Autodesk Fusion 360 part; units mm, degrees
(part 2 of 5)
  line L70 (-24.2901, -31.3342) -> (-24.2626, -31.2045)
  spline S218 degree 3 poles (-24.2626, -31.2045) (-24.2478, -31.133) (-24.1584, -30.8424) (-24.0641, -30.5586) knots 0 0 0 0 1 1 1 1
  spline S219 degree 3 poles (-23.1509, -35.7407) (-21.6967, -38.062) (-19.505, -39.4527) (-18.2798, -38.8318) knots 0 0 0 0 1 1 1 1
  spline S220 degree 3 poles (-18.2798, -38.8318) (-17.8908, -38.6347) (-17.6834, -38.3768) (-18.0232, -38.5126) knots 0 0 0 0 1 1 1 1
  spline S221 degree 3 poles (-18.0232, -38.5126) (-19.0953, -38.9415) (-20.3855, -38.1958) (-23.002, -35.6358) knots 0 0 0 0 1 1 1 1
  spline S222 degree 3 poles (-23.002, -35.6358) (-23.4422, -35.2048) (-23.4732, -35.2265) (-23.1509, -35.7407) knots 0 0 0 0 1 1 1 1
  spline S223 degree 3 poles (-20.8842, -40.3996) (-20.7556, -40.3996) (-20.6902, -40.5127) (-20.7714, -40.5939) knots 0 0 0 0 1 1 1 1
  spline S224 degree 3 poles (-20.7714, -40.5939) (-20.8663, -40.6892) (-21.0022, -40.6311) (-20.9874, -40.5014) knots 0 0 0 0 1 1 1 1
  spline S225 degree 3 poles (-20.9874, -40.5014) (-20.9781, -40.423) (-20.9547, -40.3996) (-20.8842, -40.3996) knots 0 0 0 0 1 1 1 1
  spline S226 degree 3 poles (-15.859, -39.81) (-15.7052, -39.9693) (-15.4972, -40.2273) (-15.3967, -40.3834) knots 0 0 0 0 1 1 1 1
  spline S227 degree 3 poles (-15.3967, -40.3834) (-15.0184, -40.9719) (-14.932, -41.0844) (-14.7484, -41.2302) knots 0 0 0 0 1 1 1 1
  spline S228 degree 3 poles (-14.7484, -41.2302) (-14.5557, -41.3833) (-14.2304, -41.5653) (-14.1499, -41.5653) knots 0 0 0 0 1 1 1 1
  spline S229 degree 3 poles (-14.1499, -41.5653) (-14.1251, -41.5653) (-14.2407, -41.4236) (-14.4068, -41.2499) knots 0 0 0 0 1 1 1 1
  spline S230 degree 3 poles (-14.4068, -41.2499) (-14.5726, -41.0765) (-14.7934, -40.7972) (-14.8973, -40.629) knots 0 0 0 0 1 1 1 1
  spline S231 degree 3 poles (-14.8973, -40.629) (-15.2719, -40.0226) (-15.5315, -39.7523) (-15.9388, -39.5452) knots 0 0 0 0 1 1 1 1
  spline S232 degree 3 poles (-15.9388, -39.5452) (-16.2274, -39.3987) (-16.214, -39.443) (-15.859, -39.81) knots 0 0 0 0 1 1 1 1
  spline S233 degree 3 poles (-15.6155, -38.9729) (-15.2839, -39.2931) (-14.9551, -39.4286) (-14.3803, -39.4819) knots 0 0 0 0 1 1 1 1
  spline S234 degree 3 poles (-14.3803, -39.4819) (-13.7203, -39.5431) (-12.3448, -39.3147) (-12.2268, -39.1245) knots 0 0 0 0 1 1 1 1
  spline S235 degree 3 poles (-12.2268, -39.1245) (-12.2185, -39.1111) (-12.7586, -39.106) (-13.4265, -39.1125) knots 0 0 0 0 1 1 1 1
  spline S236 degree 3 poles (-13.4265, -39.1125) (-14.7814, -39.1263) (-14.9286, -39.1111) (-15.3916, -38.9072) knots 0 0 0 0 1 1 1 1
  spline S237 degree 3 poles (-15.3916, -38.9072) (-15.5622, -38.8318) (-15.7231, -38.7613) (-15.7493, -38.7496) knots 0 0 0 0 1 1 1 1
  spline S238 degree 3 poles (-15.7493, -38.7496) (-15.849, -38.7066) (-15.7905, -38.8036) (-15.6155, -38.9729) knots 0 0 0 0 1 1 1 1
  spline S239 degree 3 poles (-13.7519, -74.1202) (-12.6942, -87.0541) (-11.8189, -97.6776) (-11.8061, -97.7278) knots 0 0 0 0 1 1 1 1
  spline S240 degree 3 poles (-11.8061, -97.7278) (-11.7607, -97.9101) (-11.4151, -97.9504) (-11.326, -97.7842) knots 0 0 0 0 1 1 1 1
  spline S241 degree 3 poles (-11.326, -97.7842) (-11.2393, -97.6222) (-11.2764, -47.9849) (-11.3638, -47.8422) knots 0 0 0 0 1 1 1 1
  spline S242 degree 3 poles (-11.3638, -47.8422) (-11.5103, -47.6017) (-11.8199, -47.4865) (-12.0768, -47.5766) knots 0 0 0 0 1 1 1 1
  spline S243 degree 3 poles (-12.0768, -47.5766) (-12.3517, -47.6733) (-15.5192, -49.7374) (-15.6048, -49.8756) knots 0 0 0 0 1 1 1 1
  spline S244 degree 3 poles (-15.6048, -49.8756) (-15.7235, -50.0676) (-15.7985, -49.0845) (-13.7519, -74.1202) knots 0 0 0 0 1 1 1 1
  spline S245 degree 3 poles (-15.6055, -12.3577) (-15.59, -12.4261) (-15.5364, -12.5335) (-15.4865, -12.5964) knots 0 0 0 0 1 1 1 1
  spline S246 degree 3 poles (-15.4865, -12.5964) (-15.3713, -12.7416) (-12.158, -14.8015) (-11.9657, -14.8538) knots 0 0 0 0 1 1 1 1
  spline S247 degree 3 poles (-11.9657, -14.8538) (-11.6961, -14.9264) (-11.3941, -14.7857) (-11.273, -14.5312) knots 0 0 0 0 1 1 1 1
  spline S248 degree 3 poles (-11.273, -14.5312) (-11.2159, -14.4104) (-11.2111, -12.4203) (-11.2111, 10.4615) knots 0 0 0 0 1 1 1 1
  line L71 (-11.2111, 10.4615) -> (-11.2111, 35.3228)
  line L72 (-11.2111, 35.3228) -> (-11.3115, 35.4023)
  spline S249 degree 3 poles (-11.3115, 35.4023) (-11.4347, 35.4989) (-11.5578, 35.5031) (-11.6675, 35.4143) knots 0 0 0 0 1 1 1 1
  spline S250 degree 3 poles (-11.6675, 35.4143) (-11.748, 35.349) (-11.7989, 34.7477) (-13.6755, 11.729) knots 0 0 0 0 1 1 1 1
  spline S251 degree 3 poles (-13.6755, 11.729) (-14.7346, -1.2609) (-15.6082, -11.9666) (-15.6172, -12.0612) knots 0 0 0 0 1 1 1 1
  spline S252 degree 3 poles (-15.6172, -12.0612) (-15.6261, -12.1558) (-15.6206, -12.2892) (-15.6055, -12.3577) knots 0 0 0 0 1 1 1 1
  spline S253 degree 3 poles (-15.1442, -35.3867) (-14.6259, -35.8559) (-13.8018, -36.1269) (-13.1434, -36.0447) knots 0 0 0 0 1 1 1 1
  spline S254 degree 3 poles (-13.1434, -36.0447) (-12.8686, -36.0103) (-12.8755, -35.9856) (-13.1888, -35.8765) knots 0 0 0 0 1 1 1 1
  spline S255 degree 3 poles (-13.1888, -35.8765) (-13.4503, -35.7854) (-15.2412, -35.1494) (-15.329, -35.1164) knots 0 0 0 0 1 1 1 1
  spline S256 degree 3 poles (-15.329, -35.1164) (-15.4404, -35.0744) (-15.3609, -35.191) (-15.1442, -35.3867) knots 0 0 0 0 1 1 1 1
  spline S257 degree 3 poles (-10.2752, -41.426) (-10.171, -41.0755) (-9.569, -40.3411) (-9.3878, -40.3432) knots 0 0 0 0 1 1 1 1
  spline S258 degree 3 poles (-9.3878, -40.3432) (-9.0524, -40.3473) (-8.8275, -40.6087) (-8.8797, -40.9341) knots 0 0 0 0 1 1 1 1
  spline S259 degree 3 poles (-8.8797, -40.9341) (-8.9637, -41.4597) (-9.1202, -41.6488) (-9.5436, -41.7376) knots 0 0 0 0 1 1 1 1
  spline S260 degree 3 poles (-9.5436, -41.7376) (-9.686, -41.7675) (-9.8573, -41.8256) (-9.9243, -41.8673) knots 0 0 0 0 1 1 1 1
  spline S261 degree 3 poles (-9.9243, -41.8673) (-10.3061, -42.1032) (-10.43, -41.9477) (-10.2752, -41.426) knots 0 0 0 0 1 1 1 1
  spline S262 degree 3 poles (-4.9222, -79.0378) (-4.4427, -81.601) (-2.4986, -83.2055) (0.1206, -83.1997) knots 0 0 0 0 1 1 1 1
  spline S263 degree 3 poles (0.1206, -83.1997) (3.6706, -83.1918) (5.9848, -79.9675) (4.9739, -76.4378) knots 0 0 0 0 1 1 1 1
  spline S264 degree 3 poles (4.9739, -76.4378) (3.682, -71.9251) (-2.9984, -71.6857) (-4.6573, -76.0925) knots 0 0 0 0 1 1 1 1
  spline S265 degree 3 poles (-4.6573, -76.0925) (-4.9524, -76.8767) (-5.0738, -78.2264) (-4.9222, -79.0378) knots 0 0 0 0 1 1 1 1
  spline S266 degree 3 poles (-4.9242, -57.9033) (-4.4138, -60.7987) (-1.6762, -62.6382) (1.1996, -62.0184) knots 0 0 0 0 1 1 1 1
  spline S267 degree 3 poles (1.1996, -62.0184) (5.118, -61.174) (6.5392, -56.3479) (3.7927, -53.212) knots 0 0 0 0 1 1 1 1
  spline S268 degree 3 poles (3.7927, -53.212) (3.6317, -53.028) (3.479, -52.8777) (3.4529, -52.8777) knots 0 0 0 0 1 1 1 1
  spline S269 degree 3 poles (3.4529, -52.8777) (3.4102, -52.8777) (3.1217, -53.1625) (2.2081, -54.1063) knots 0 0 0 0 1 1 1 1
  line L73 (2.2081, -54.1063) -> (1.8882, -54.4365)
  line L74 (1.8882, -54.4365) -> (2.0781, -54.6649)
  spline S270 degree 3 poles (2.0781, -54.6649) (3.8804, -56.8305) (2.7553, -59.6901) (0.1014, -59.6901) knots 0 0 0 0 1 1 1 1
  spline S271 degree 3 poles (0.1014, -59.6901) (-2.5523, -59.6901) (-3.6774, -56.8305) (-1.8757, -54.6656) knots 0 0 0 0 1 1 1 1
  line L75 (-1.8757, -54.6656) -> (-1.6865, -54.4379)
  line L76 (-1.6865, -54.4379) -> (-1.798, -54.3172)
  spline S272 degree 3 poles (-1.798, -54.3172) (-1.8592, -54.2504) (-2.2094, -53.8803) (-2.576, -53.4944) knots 0 0 0 0 1 1 1 1
  line L77 (-2.576, -53.4944) -> (-3.2426, -52.7924)
  line L78 (-3.2426, -52.7924) -> (-3.537, -53.1061)
  spline S273 degree 3 poles (-3.537, -53.1061) (-4.1995, -53.8119) (-4.6312, -54.613) (-4.8554, -55.553) knots 0 0 0 0 1 1 1 1
  spline S274 degree 3 poles (-4.8554, -55.553) (-4.9762, -56.06) (-5.0154, -57.3877) (-4.9242, -57.9033) knots 0 0 0 0 1 1 1 1
  spline S275 degree 3 poles (-4.9222, -38.4889) (-4.4427, -41.0521) (-2.4986, -42.6566) (0.1206, -42.6508) knots 0 0 0 0 1 1 1 1
  spline S276 degree 3 poles (0.1206, -42.6508) (3.6706, -42.6429) (5.9848, -39.4186) (4.9739, -35.8889) knots 0 0 0 0 1 1 1 1
  spline S277 degree 3 poles (4.9739, -35.8889) (3.682, -31.3762) (-2.9984, -31.1371) (-4.6573, -35.5439) knots 0 0 0 0 1 1 1 1
  spline S278 degree 3 poles (-4.6573, -35.5439) (-4.9524, -36.3278) (-5.0738, -37.6775) (-4.9222, -38.4889) knots 0 0 0 0 1 1 1 1
  spline S279 degree 3 poles (-4.9222, -15.6346) (-4.4427, -18.1978) (-2.4986, -19.8027) (0.1206, -19.7968) knots 0 0 0 0 1 1 1 1
  spline S280 degree 3 poles (0.1206, -19.7968) (3.6706, -19.7889) (5.9848, -16.5646) (4.9739, -13.0346) knots 0 0 0 0 1 1 1 1
  spline S281 degree 3 poles (4.9739, -13.0346) (3.682, -8.5222) (-2.9984, -8.2828) (-4.6573, -12.6896) knots 0 0 0 0 1 1 1 1
  spline S282 degree 3 poles (-4.6573, -12.6896) (-4.9524, -13.4738) (-5.0738, -14.8235) (-4.9222, -15.6346) knots 0 0 0 0 1 1 1 1
  spline S283 degree 3 poles (-4.9222, 3.474) (-4.4427, 0.9108) (-2.4986, -0.6937) (0.1206, -0.6879) knots 0 0 0 0 1 1 1 1
  spline S284 degree 3 poles (0.1206, -0.6879) (3.6706, -0.68) (5.9848, 2.5443) (4.9739, 6.074) knots 0 0 0 0 1 1 1 1
  spline S285 degree 3 poles (4.9739, 6.074) (3.682, 10.5867) (-2.9984, 10.8258) (-4.6573, 6.419) knots 0 0 0 0 1 1 1 1
  spline S286 degree 3 poles (-4.6573, 6.419) (-4.9524, 5.6351) (-5.0738, 4.2854) (-4.9222, 3.474) knots 0 0 0 0 1 1 1 1
  spline S287 degree 3 poles (-4.9242, 24.6085) (-4.4138, 21.7131) (-1.6762, 19.8736) (1.1996, 20.4934) knots 0 0 0 0 1 1 1 1
  spline S288 degree 3 poles (1.1996, 20.4934) (5.118, 21.3378) (6.5392, 26.1639) (3.7927, 29.2998) knots 0 0 0 0 1 1 1 1
  spline S289 degree 3 poles (3.7927, 29.2998) (3.6317, 29.4835) (3.479, 29.6341) (3.4529, 29.6341) knots 0 0 0 0 1 1 1 1
  spline S290 degree 3 poles (3.4529, 29.6341) (3.4102, 29.6341) (3.1217, 29.3493) (2.2081, 28.4055) knots 0 0 0 0 1 1 1 1
  line L79 (2.2081, 28.4055) -> (1.8882, 28.0753)
  line L80 (1.8882, 28.0753) -> (2.0781, 27.8469)
  spline S291 degree 3 poles (2.0781, 27.8469) (3.8804, 25.6813) (2.7553, 22.8217) (0.1014, 22.8217) knots 0 0 0 0 1 1 1 1
  spline S292 degree 3 poles (0.1014, 22.8217) (-2.5523, 22.8217) (-3.6774, 25.6813) (-1.8757, 27.8462) knots 0 0 0 0 1 1 1 1
  line L81 (-1.8757, 27.8462) -> (-1.6865, 28.0739)
  line L82 (-1.6865, 28.0739) -> (-1.798, 28.1947)
  spline S293 degree 3 poles (-1.798, 28.1947) (-1.8592, 28.261) (-2.2094, 28.6315) (-2.576, 29.0174) knots 0 0 0 0 1 1 1 1
  line L83 (-2.576, 29.0174) -> (-3.2426, 29.7194)
  line L84 (-3.2426, 29.7194) -> (-3.537, 29.4057)
  spline S294 degree 3 poles (-3.537, 29.4057) (-4.1995, 28.6999) (-4.6312, 27.8988) (-4.8554, 26.9588) knots 0 0 0 0 1 1 1 1
  spline S295 degree 3 poles (-4.8554, 26.9588) (-4.9762, 26.4518) (-5.0154, 25.1241) (-4.9242, 24.6085) knots 0 0 0 0 1 1 1 1
  spline S296 degree 3 poles (-4.9252, 32.6341) (-4.5713, 31.0117) (-3.1164, 29.9402) (-1.5187, 30.126) knots 0 0 0 0 1 1 1 1
  spline S297 degree 3 poles (-1.5187, 30.126) (-0.1704, 30.2828) (0.499, 30.9728) (1.1549, 32.8828) knots 0 0 0 0 1 1 1 1
  spline S298 degree 3 poles (1.1549, 32.8828) (1.6144, 34.2208) (1.9742, 34.5482) (2.6239, 34.2194) knots 0 0 0 0 1 1 1 1
  spline S299 degree 3 poles (2.6239, 34.2194) (3.3851, 33.8342) (3.0343, 32.424) (2.1768, 32.424) knots 0 0 0 0 1 1 1 1
  line L85 (2.1768, 32.424) -> (2.0506, 32.424)
  line L86 (2.0506, 32.424) -> (2.0506, 31.2545)
  line L87 (2.0506, 31.2545) -> (2.0506, 30.085)
  line L88 (2.0506, 30.085) -> (2.3275, 30.1108)
  spline S300 degree 3 poles (2.3275, 30.1108) (4.2423, 30.2897) (5.3419, 31.6934) (5.1765, 33.7479) knots 0 0 0 0 1 1 1 1
  spline S301 degree 3 poles (5.1765, 33.7479) (4.9292, 36.8191) (0.8178, 37.7501) (-0.5377, 35.0418) knots 0 0 0 0 1 1 1 1
  spline S302 degree 3 poles (-0.5377, 35.0418) (-0.6794, 34.7581) (-0.8094, 34.3948) (-0.9821, 33.7998) knots 0 0 0 0 1 1 1 1
  spline S303 degree 3 poles (-0.9821, 33.7998) (-1.2934, 32.7256) (-1.4929, 32.4529) (-1.9634, 32.4563) knots 0 0 0 0 1 1 1 1
  spline S304 degree 3 poles (-1.9634, 32.4563) (-3.0624, 32.4649) (-3.1387, 34.2094) (-2.0484, 34.3911) knots 0 0 0 0 1 1 1 1
  line L89 (-2.0484, 34.3911) -> (-1.886, 34.4179)
  line L90 (-1.886, 34.4179) -> (-1.886, 35.5285)
  line L91 (-1.886, 35.5285) -> (-1.886, 36.6388)
  line L92 (-1.886, 36.6388) -> (-2.1454, 36.6147)
  spline S305 degree 3 poles (-2.1454, 36.6147) (-4.129, 36.4304) (-5.3669, 34.658) (-4.9252, 32.6341) knots 0 0 0 0 1 1 1 1
  line L93 (0.1189, -99.0827) -> (4.9168, -99.0827)
  line L94 (4.9168, -99.0827) -> (4.9161, -97.0478)
  spline S306 degree 3 poles (4.9161, -97.0478) (4.9157, -95.9282) (4.8989, -94.8097) (4.8783, -94.5617) knots 0 0 0 0 1 1 1 1
  spline S307 degree 3 poles (4.8783, -94.5617) (4.6598, -91.9245) (1.8174, -91.0416) (0.1781, -93.1012) knots 0 0 0 0 1 1 1 1
  line L95 (0.1781, -93.1012) -> (-0.017, -93.3468)
  line L96 (-0.017, -93.3468) -> (-0.3303, -93.0304)
  spline S308 degree 3 poles (-0.3303, -93.0304) (-1.5407, -91.8086) (-3.7197, -92.2936) (-4.4275, -93.9425) knots 0 0 0 0 1 1 1 1
  spline S309 degree 3 poles (-4.4275, -93.9425) (-4.6642, -94.4932) (-4.6521, -94.3474) (-4.6662, -96.8184) knots 0 0 0 0 1 1 1 1
  line L97 (-4.6662, -96.8184) -> (-4.6793, -99.0827)
  line L98 (-4.6793, -99.0827) -> (0.1189, -99.0827)
  line L99 (0.1206, -91.3629) -> (4.9168, -91.3629)
  line L100 (4.9168, -91.3629) -> (4.9168, -90.1786)
  line L101 (4.9168, -90.1786) -> (4.9168, -88.994)
  line L102 (4.9168, -88.994) -> (3.1726, -88.984)
  line L103 (3.1726, -88.984) -> (1.428, -88.9741)
  line L104 (1.428, -88.9741) -> (3.1629, -87.7854)
  line L105 (3.1629, -87.7854) -> (4.8979, -86.5963)
  line L106 (4.8979, -86.5963) -> (4.9078, -85.1197)
  spline S310 degree 3 poles (4.9078, -85.1197) (4.914, -84.1972) (4.904, -83.6427) (4.881, -83.6427) knots 0 0 0 0 1 1 1 1
  spline S311 degree 3 poles (4.881, -83.6427) (4.8611, -83.6427) (4.0655, -84.2102) (3.1131, -84.9033) knots 0 0 0 0 1 1 1 1
  spline S312 degree 3 poles (3.1131, -84.9033) (2.161, -85.5967) (1.3719, -86.1643) (1.3602, -86.1646) knots 0 0 0 0 1 1 1 1
  spline S313 degree 3 poles (1.3602, -86.1646) (1.3486, -86.165) (1.3162, -86.0762) (1.2884, -85.9675) knots 0 0 0 0 1 1 1 1
  spline S314 degree 3 poles (1.2884, -85.9675) (1.0514, -85.0433) (0.2806, -84.2983) (-0.6908, -84.0544) knots 0 0 0 0 1 1 1 1
  spline S315 degree 3 poles (-0.6908, -84.0544) (-2.3731, -83.6327) (-3.9494, -84.418) (-4.4654, -85.9352) knots 0 0 0 0 1 1 1 1
  spline S316 degree 3 poles (-4.4654, -85.9352) (-4.6683, -86.532) (-4.6759, -86.6441) (-4.6759, -89.0931) knots 0 0 0 0 1 1 1 1
  line L107 (-4.6759, -89.0931) -> (-4.6759, -91.3629)
  line L108 (-4.6759, -91.3629) -> (0.1206, -91.3629)
  line L109 (0.1206, -71.7572) -> (4.9168, -71.7572)
  line L110 (4.9168, -71.7572) -> (4.9168, -70.5726)
  line L111 (4.9168, -70.5726) -> (4.9168, -69.3881)
  line L112 (4.9168, -69.3881) -> (2.1183, -69.3784)
  line L113 (2.1183, -69.3784) -> (-0.6805, -69.3684)
  line L114 (-0.6805, -69.3684) -> (2.1183, -67.5348)
  line L115 (2.1183, -67.5348) -> (4.9168, -65.7008)
  line L116 (4.9168, -65.7008) -> (4.9168, -64.4677)
  line L117 (4.9168, -64.4677) -> (4.9168, -63.2346)
  line L118 (4.9168, -63.2346) -> (0.1206, -63.2346)
  line L119 (0.1206, -63.2346) -> (-4.6759, -63.2346)
  line L120 (-4.6759, -63.2346) -> (-4.6759, -64.4192)
  line L121 (-4.6759, -64.4192) -> (-4.6759, -65.6038)
  line L122 (-4.6759, -65.6038) -> (-1.8964, -65.6135)
  line L123 (-1.8964, -65.6135) -> (0.8832, -65.6234)
  line L124 (0.8832, -65.6234) -> (-1.8964, -67.4364)
  line L125 (-1.8964, -67.4364) -> (-4.6759, -69.2494)
  line L126 (-4.6759, -69.2494) -> (-4.6759, -70.5032)
  line L127 (-4.6759, -70.5032) -> (-4.6759, -71.7572)
  line L128 (-4.6759, -71.7572) -> (0.1206, -71.7572)
  line L129 (0.1206, -52.1898) -> (4.9168, -52.1898)
  line L130 (4.9168, -52.1898) -> (4.9168, -51.0052)
  line L131 (4.9168, -51.0052) -> (4.9168, -49.8203)
  line L132 (4.9168, -49.8203) -> (3.0061, -49.8203)
  line L133 (3.0061, -49.8203) -> (1.0951, -49.8203)
  line L134 (1.0951, -49.8203) -> (1.0951, -47.9667)
  line L135 (1.0951, -47.9667) -> (1.0951, -46.1131)
  line L136 (1.0951, -46.1131) -> (3.0061, -46.1131)
  line L137 (3.0061, -46.1131) -> (4.9168, -46.1131)
  line L138 (4.9168, -46.1131) -> (4.9168, -44.9474)
  line L139 (4.9168, -44.9474) -> (4.9168, -43.7821)
  line L140 (4.9168, -43.7821) -> (0.1206, -43.7821)
  line L141 (0.1206, -43.7821) -> (-4.6759, -43.7821)
  line L142 (-4.6759, -43.7821) -> (-4.6759, -44.9474)
  line L143 (-4.6759, -44.9474) -> (-4.6759, -46.1131)
  line L144 (-4.6759, -46.1131) -> (-2.803, -46.1131)
  line L145 (-2.803, -46.1131) -> (-0.9305, -46.1131)
  line L146 (-0.9305, -46.1131) -> (-0.9305, -47.9667)
  line L147 (-0.9305, -47.9667) -> (-0.9305, -49.8203)
  line L148 (-0.9305, -49.8203) -> (-2.803, -49.8203)
  line L149 (-2.803, -49.8203) -> (-4.6759, -49.8203)
  line L150 (-4.6759, -49.8203) -> (-4.6759, -51.0052)
  line L151 (-4.6759, -51.0052) -> (-4.6759, -52.1898)
  line L152 (-4.6759, -52.1898) -> (0.1206, -52.1898)
  line L153 (0.1206, -27.96) -> (4.9168, -27.96)
  line L154 (4.9168, -27.96) -> (4.9168, -26.7754)
  line L155 (4.9168, -26.7754) -> (4.9168, -25.5912)
  line L156 (4.9168, -25.5912) -> (3.1726, -25.5812)
  line L157 (3.1726, -25.5812) -> (1.428, -25.5712)
  line L158 (1.428, -25.5712) -> (3.1629, -24.3821)
  line L159 (3.1629, -24.3821) -> (4.8979, -23.1934)
  line L160 (4.8979, -23.1934) -> (4.9078, -21.7165)
  spline S317 degree 3 poles (4.9078, -21.7165) (4.914, -20.7943) (4.904, -20.2398) (4.881, -20.2398) knots 0 0 0 0 1 1 1 1
  spline S318 degree 3 poles (4.881, -20.2398) (4.8611, -20.2398) (4.0655, -20.807) (3.1131, -21.5005) knots 0 0 0 0 1 1 1 1
  spline S319 degree 3 poles (3.1131, -21.5005) (2.161, -22.1935) (1.3719, -22.7611) (1.3602, -22.7614) knots 0 0 0 0 1 1 1 1
  spline S320 degree 3 poles (1.3602, -22.7614) (1.3486, -22.7621) (1.3162, -22.6734) (1.2884, -22.5647) knots 0 0 0 0 1 1 1 1
  spline S321 degree 3 poles (1.2884, -22.5647) (1.0514, -21.6404) (0.2806, -20.8951) (-0.6908, -20.6516) knots 0 0 0 0 1 1 1 1
  spline S322 degree 3 poles (-0.6908, -20.6516) (-2.3731, -20.2295) (-3.9494, -21.0151) (-4.4654, -22.5323) knots 0 0 0 0 1 1 1 1
  spline S323 degree 3 poles (-4.4654, -22.5323) (-4.6683, -23.1291) (-4.6759, -23.2409) (-4.6759, -25.6902) knots 0 0 0 0 1 1 1 1
  line L161 (-4.6759, -25.6902) -> (-4.6759, -27.96)
  line L162 (-4.6759, -27.96) -> (0.1206, -27.96)
  line L163 (0.1189, -8.3544) -> (4.9168, -8.3544)
  line L164 (4.9168, -8.3544) -> (4.9161, -6.3192)
  spline S324 degree 3 poles (4.9161, -6.3192) (4.9157, -5.1999) (4.8989, -4.081) (4.8783, -3.833) knots 0 0 0 0 1 1 1 1
  spline S325 degree 3 poles (4.8783, -3.833) (4.6598, -1.1959) (1.8174, -0.313) (0.1781, -2.3729) knots 0 0 0 0 1 1 1 1
  line L165 (0.1781, -2.3729) -> (-0.017, -2.6182)
  line L166 (-0.017, -2.6182) -> (-0.3303, -2.3017)
  spline S326 degree 3 poles (-0.3303, -2.3017) (-1.5407, -1.08) (-3.7197, -1.565) (-4.4275, -3.2139) knots 0 0 0 0 1 1 1 1
  spline S327 degree 3 poles (-4.4275, -3.2139) (-4.6642, -3.7646) (-4.6521, -3.6191) (-4.6662, -6.0897) knots 0 0 0 0 1 1 1 1
  line L167 (-4.6662, -6.0897) -> (-4.6793, -8.3544)
  line L168 (-4.6793, -8.3544) -> (0.1189, -8.3544)
  line L169 (-3.644, 9.6464) -> (-2.6121, 9.6464)
  line L170 (-2.6121, 9.6464) -> (-2.6121, 10.7164)
  line L171 (-2.6121, 10.7164) -> (-2.6121, 11.7865)
  line L172 (-2.6121, 11.7865) -> (1.1525, 11.7865)
  line L173 (1.1525, 11.7865) -> (4.9168, 11.7865)
  line L174 (4.9168, 11.7865) -> (4.9168, 12.9711)
  line L175 (4.9168, 12.9711) -> (4.9168, 14.156)
  line L176 (4.9168, 14.156) -> (1.1525, 14.156)
  line L177 (1.1525, 14.156) -> (-2.6121, 14.156)
  line L178 (-2.6121, 14.156) -> (-2.6121, 15.2453)
  line L179 (-2.6121, 15.2453) -> (-2.6121, 16.3343)
  line L180 (-2.6121, 16.3343) -> (-3.644, 16.3343)
  line L181 (-3.644, 16.3343) -> (-4.6759, 16.3343)
  line L182 (-4.6759, 16.3343) -> (-4.6759, 12.9903)
  line L183 (-4.6759, 12.9903) -> (-4.6759, 9.6464)
  line L184 (-4.6759, 9.6464) -> (-3.644, 9.6464)
  line L185 (0.1206, 16.9458) -> (4.9168, 16.9458)
  line L186 (4.9168, 16.9458) -> (4.9168, 18.1304)
  line L187 (4.9168, 18.1304) -> (4.9168, 19.3154)
  line L188 (4.9168, 19.3154) -> (0.1206, 19.3154)
  line L189 (0.1206, 19.3154) -> (-4.6759, 19.3154)
  line L190 (-4.6759, 19.3154) -> (-4.6759, 18.1304)
  line L191 (-4.6759, 18.1304) -> (-4.6759, 16.9458)
  line L192 (-4.6759, 16.9458) -> (0.1206, 16.9458)
  spline S328 degree 3 poles (-4.4272, -77.1529) (-3.5357, -72.5222) (3.3672, -72.2945) (4.5343, -76.8571) knots 0 0 0 0 1 1 1 1
  spline S329 degree 3 poles (4.5343, -76.8571) (5.2993, -79.8489) (3.1846, -82.5778) (0.1014, -82.5778) knots 0 0 0 0 1 1 1 1
  spline S330 degree 3 poles (0.1014, -82.5778) (-2.8794, -82.5778) (-4.9861, -80.0545) (-4.4272, -77.1529) knots 0 0 0 0 1 1 1 1
  spline S331 degree 3 poles (-4.4833, -56.32) (-4.3832, -55.3449) (-4.012, -54.4472) (-3.45, -53.8205) knots 0 0 0 0 1 1 1 1
  line L193 (-3.45, -53.8205) -> (-3.2502, -53.5976)
  line L194 (-3.2502, -53.5976) -> (-2.8202, -54.0262)
  line L195 (-2.8202, -54.0262) -> (-2.3903, -54.4551)
  line L196 (-2.3903, -54.4551) -> (-2.5193, -54.6346)
  spline S332 degree 3 poles (-2.5193, -54.6346) (-3.4844, -55.9781) (-3.4603, -58.0254) (-2.4656, -59.2076) knots 0 0 0 0 1 1 1 1
  spline S333 degree 3 poles (-2.4656, -59.2076) (-1.1933, -60.7193) (1.396, -60.7193) (2.6683, -59.2076) knots 0 0 0 0 1 1 1 1
  spline S334 degree 3 poles (2.6683, -59.2076) (3.6589, -58.0305) (3.6913, -55.9551) (2.7385, -54.6893) knots 0 0 0 0 1 1 1 1
  line L197 (2.7385, -54.6893) -> (2.592, -54.4943)
  line L198 (2.592, -54.4943) -> (3.0309, -54.0589)
  line L199 (3.0309, -54.0589) -> (3.4697, -53.6231)
  line L200 (3.4697, -53.6231) -> (3.6053, -53.7758)
  spline S335 degree 3 poles (3.6053, -53.7758) (5.6553, -56.0927) (4.7868, -59.9516) (1.9491, -61.1327) knots 0 0 0 0 1 1 1 1
  spline S336 degree 3 poles (1.9491, -61.1327) (-1.4014, -62.5275) (-4.8551, -59.9436) (-4.4833, -56.32) knots 0 0 0 0 1 1 1 1
  spline S337 degree 3 poles (-4.4272, -36.604) (-3.5357, -31.9733) (3.3672, -31.7456) (4.5343, -36.3082) knots 0 0 0 0 1 1 1 1
  spline S338 degree 3 poles (4.5343, -36.3082) (5.2993, -39.3) (3.1846, -42.0289) (0.1014, -42.0289) knots 0 0 0 0 1 1 1 1
  spline S339 degree 3 poles (0.1014, -42.0289) (-2.8794, -42.0289) (-4.9861, -39.5056) (-4.4272, -36.604) knots 0 0 0 0 1 1 1 1
  spline S340 degree 3 poles (-4.4272, -13.75) (-3.5357, -9.1193) (3.3672, -8.8916) (4.5343, -13.4542) knots 0 0 0 0 1 1 1 1
  spline S341 degree 3 poles (4.5343, -13.4542) (5.2993, -16.4456) (3.1846, -19.175) (0.1014, -19.175) knots 0 0 0 0 1 1 1 1
  spline S342 degree 3 poles (0.1014, -19.175) (-2.8794, -19.175) (-4.9861, -16.6517) (-4.4272, -13.75) knots 0 0 0 0 1 1 1 1
  spline S343 degree 3 poles (-4.4272, 5.3589) (-3.5357, 9.9896) (3.3672, 10.2173) (4.5343, 5.6547) knots 0 0 0 0 1 1 1 1
  spline S344 degree 3 poles (4.5343, 5.6547) (5.2993, 2.663) (3.1846, -0.066) (0.1014, -0.066) knots 0 0 0 0 1 1 1 1
  spline S345 degree 3 poles (0.1014, -0.066) (-2.8794, -0.066) (-4.9861, 2.4573) (-4.4272, 5.3589) knots 0 0 0 0 1 1 1 1
  spline S346 degree 3 poles (-4.4833, 26.1914) (-4.3832, 27.1669) (-4.012, 28.0646) (-3.45, 28.6913) knots 0 0 0 0 1 1 1 1
  line L201 (-3.45, 28.6913) -> (-3.2502, 28.9142)
  line L202 (-3.2502, 28.9142) -> (-2.8202, 28.4856)
  line L203 (-2.8202, 28.4856) -> (-2.3903, 28.0567)
  line L204 (-2.3903, 28.0567) -> (-2.5193, 27.8772)
  spline S347 degree 3 poles (-2.5193, 27.8772) (-3.4844, 26.5337) (-3.4603, 24.4864) (-2.4656, 23.3042) knots 0 0 0 0 1 1 1 1
  spline S348 degree 3 poles (-2.4656, 23.3042) (-1.1933, 21.7926) (1.396, 21.7926) (2.6683, 23.3042) knots 0 0 0 0 1 1 1 1
  spline S349 degree 3 poles (2.6683, 23.3042) (3.6589, 24.4813) (3.6913, 26.5567) (2.7385, 27.8225) knots 0 0 0 0 1 1 1 1
  line L205 (2.7385, 27.8225) -> (2.592, 28.0175)
  line L206 (2.592, 28.0175) -> (3.0309, 28.453)
  line L207 (3.0309, 28.453) -> (3.4697, 28.8887)
  line L208 (3.4697, 28.8887) -> (3.6053, 28.736)
  spline S350 degree 3 poles (3.6053, 28.736) (5.6553, 26.4188) (4.7868, 22.5603) (1.9491, 21.3791) knots 0 0 0 0 1 1 1 1
  spline S351 degree 3 poles (1.9491, 21.3791) (-1.4014, 19.9844) (-4.8551, 22.5682) (-4.4833, 26.1914) knots 0 0 0 0 1 1 1 1
  spline S352 degree 3 poles (-4.4062, 34.2201) (-4.1665, 35.0831) (-3.5161, 35.7459) (-2.7019, 35.9557) knots 0 0 0 0 1 1 1 1
  spline S353 degree 3 poles (-2.7019, 35.9557) (-2.3167, 36.0551) (-2.3445, 36.0943) (-2.3445, 35.4529) knots 0 0 0 0 1 1 1 1
  line L209 (-2.3445, 35.4529) -> (-2.3445, 34.8891)
  line L210 (-2.3445, 34.8891) -> (-2.5557, 34.7787)
  spline S354 degree 3 poles (-2.5557, 34.7787) (-3.0576, 34.5166) (-3.3, 34.0681) (-3.3, 33.4015) knots 0 0 0 0 1 1 1 1
  spline S355 degree 3 poles (-3.3, 33.4015) (-3.3, 32.4412) (-2.8226, 31.908) (-1.9624, 31.908) knots 0 0 0 0 1 1 1 1
  spline S356 degree 3 poles (-1.9624, 31.908) (-1.1761, 31.908) (-0.9512, 32.1687) (-0.5112, 33.5886) knots 0 0 0 0 1 1 1 1
  spline S357 degree 3 poles (-0.5112, 33.5886) (-0.0166, 35.1856) (0.4175, 35.7315) (1.3909, 35.9805) knots 0 0 0 0 1 1 1 1
  spline S358 degree 3 poles (1.3909, 35.9805) (2.6191, 36.2945) (3.8983, 35.6933) (4.4435, 34.5451) knots 0 0 0 0 1 1 1 1
  spline S359 degree 3 poles (4.4435, 34.5451) (5.1954, 32.9619) (4.2701, 30.9281) (2.7034, 30.72) knots 0 0 0 0 1 1 1 1
  line L211 (2.7034, 30.72) -> (2.5091, 30.6942)
  line L212 (2.5091, 30.6942) -> (2.5091, 31.2865)
  line L213 (2.5091, 31.2865) -> (2.5091, 31.8788)
  line L214 (2.5091, 31.8788) -> (2.6989, 31.9576)
  spline S360 degree 3 poles (2.6989, 31.9576) (4.0459, 32.5172) (3.727, 34.8086) (2.2951, 34.8637) knots 0 0 0 0 1 1 1 1
  spline S361 degree 3 poles (2.2951, 34.8637) (1.5157, 34.8932) (1.2123, 34.5692) (0.7146, 33.1738) knots 0 0 0 0 1 1 1 1
  spline S362 degree 3 poles (0.7146, 33.1738) (0.0811, 31.3983) (-0.4552, 30.8228) (-1.584, 30.7059) knots 0 0 0 0 1 1 1 1
  spline S363 degree 3 poles (-1.584, 30.7059) (-3.4789, 30.5095) (-4.9335, 32.3211) (-4.4062, 34.2201) knots 0 0 0 0 1 1 1 1
  spline S364 degree 3 poles (-4.0905, -94.5173) (-3.4607, -92.7349) (-1.1661, -92.414) (-0.1848, -93.9711) knots 0 0 0 0 1 1 1 1
  spline S365 degree 3 poles (-0.1848, -93.9711) (-0.0314, -94.2143) (0.0487, -94.2105) (0.2042, -93.9522) knots 0 0 0 0 1 1 1 1
  spline S366 degree 3 poles (0.2042, -93.9522) (1.3324, -92.0776) (3.748, -92.2062) (4.3283, -94.172) knots 0 0 0 0 1 1 1 1
  spline S367 degree 3 poles (4.3283, -94.172) (4.3881, -94.3756) (4.3974, -94.6277) (4.4101, -96.4362) knots 0 0 0 0 1 1 1 1
  line L215 (4.4101, -96.4362) -> (4.4242, -98.4714)
  line L216 (4.4242, -98.4714) -> (0.1017, -98.4714)
  line L217 (0.1017, -98.4714) -> (-4.2212, -98.4714)
  line L218 (-4.2212, -98.4714) -> (-4.2095, -96.6464)
  line L219 (-4.2095, -96.6464) -> (-4.1981, -94.8214)
  line L220 (-4.1981, -94.8214) -> (-4.0905, -94.5173)
  spline S368 degree 3 poles (-4.1242, -86.5856) (-3.7685, -85.3064) (-2.8202, -84.5852) (-1.5036, -84.5924) knots 0 0 0 0 1 1 1 1
  spline S369 degree 3 poles (-1.5036, -84.5924) (-0.1456, -84.5996) (0.6599, -85.2951) (0.9275, -86.6916) knots 0 0 0 0 1 1 1 1
  spline S370 degree 3 poles (0.9275, -86.6916) (0.9891, -87.0118) (1.0032, -87.0441) (1.0813, -87.0441) knots 0 0 0 0 1 1 1 1
  spline S371 degree 3 poles (1.0813, -87.0441) (1.1336, -87.0441) (1.7947, -86.588) (2.7698, -85.8784) knots 0 0 0 0 1 1 1 1
  spline S372 degree 3 poles (2.7698, -85.8784) (3.651, -85.2377) (4.383, -84.7131) (4.396, -84.7131) knots 0 0 0 0 1 1 1 1
  spline S373 degree 3 poles (4.396, -84.7131) (4.4094, -84.7131) (4.4201, -85.045) (4.4201, -85.4506) knots 0 0 0 0 1 1 1 1
  line L221 (4.4201, -85.4506) -> (4.4201, -86.1884)
  line L222 (4.4201, -86.1884) -> (2.7203, -87.352)
  line L223 (2.7203, -87.352) -> (1.0204, -88.5156)
  line L224 (1.0204, -88.5156) -> (1.0194, -89.0601)
  line L225 (1.0194, -89.0601) -> (1.0187, -89.6049)
  line L226 (1.0187, -89.6049) -> (2.7192, -89.6049)
  line L227 (2.7192, -89.6049) -> (4.4201, -89.6049)
  line L228 (4.4201, -89.6049) -> (4.4201, -90.1779)
  line L229 (4.4201, -90.1779) -> (4.4201, -90.7513)
  line L230 (4.4201, -90.7513) -> (0.0989, -90.7513)
  line L231 (0.0989, -90.7513) -> (-4.2222, -90.7513)
  line L232 (-4.2222, -90.7513) -> (-4.2078, -88.7928)
  spline S374 degree 3 poles (-4.2078, -88.7928) (-4.1947, -87.05) (-4.1854, -86.8068) (-4.1242, -86.5856) knots 0 0 0 0 1 1 1 1
  line L233 (-0.8937, -67.4939) -> (2.4296, -65.3176)
  line L234 (2.4296, -65.3176) -> (2.4313, -65.155)
  line L235 (2.4313, -65.155) -> (2.4327, -64.9926)
  line L236 (2.4327, -64.9926) -> (-0.8923, -64.9926)
  line L237 (-0.8923, -64.9926) -> (-4.217, -64.9926)
  line L238 (-4.217, -64.9926) -> (-4.217, -64.4196)
  line L239 (-4.217, -64.4196) -> (-4.217, -63.8462)
  line L240 (-4.217, -63.8462) -> (0.1014, -63.8462)
  line L241 (0.1014, -63.8462) -> (4.4201, -63.8462)
  line L242 (4.4201, -63.8462) -> (4.4177, -64.5819)
  line L243 (4.4177, -64.5819) -> (4.4156, -65.3176)
  line L244 (4.4156, -65.3176) -> (1.0641, -67.5169)
  line L245 (1.0641, -67.5169) -> (-2.2871, -69.7162)
  line L246 (-2.2871, -69.7162) -> (-2.2991, -69.8576)
  line L247 (-2.2991, -69.8576) -> (-2.3108, -69.9993)
  line L248 (-2.3108, -69.9993) -> (1.0545, -69.9993)
  line L249 (1.0545, -69.9993) -> (4.4201, -69.9993)
  line L250 (4.4201, -69.9993) -> (4.4201, -70.5723)
  line L251 (4.4201, -70.5723) -> (4.4201, -71.1457)
  line L252 (4.4201, -71.1457) -> (0.1014, -71.1457)
  line L253 (0.1014, -71.1457) -> (-4.217, -71.1457)
  line L254 (-4.217, -71.1457) -> (-4.217, -70.4079)
  line L255 (-4.217, -70.4079) -> (-4.217, -69.6701)
  line L256 (-4.217, -69.6701) -> (-0.8937, -67.4939)
  line L257 (-2.3445, -50.4318) -> (-0.4717, -50.4318)
  line L258 (-0.4717, -50.4318) -> (-0.4717, -47.9667)
  line L259 (-0.4717, -47.9667) -> (-0.4717, -45.5019)
  line L260 (-0.4717, -45.5019) -> (-2.3445, -45.5019)
  line L261 (-2.3445, -45.5019) -> (-4.217, -45.5019)
  line L262 (-4.217, -45.5019) -> (-4.217, -44.9474)
  line L263 (-4.217, -44.9474) -> (-4.217, -44.3933)
  line L264 (-4.217, -44.3933) -> (0.1014, -44.3933)
  line L265 (0.1014, -44.3933) -> (4.4201, -44.3933)
  line L266 (4.4201, -44.3933) -> (4.4201, -44.9474)
  line L267 (4.4201, -44.9474) -> (4.4201, -45.5019)
  line L268 (4.4201, -45.5019) -> (2.5283, -45.5019)
  line L269 (2.5283, -45.5019) -> (0.6366, -45.5019)
  line L270 (0.6366, -45.5019) -> (0.6366, -47.9667)
  line L271 (0.6366, -47.9667) -> (0.6366, -50.4318)
  line L272 (0.6366, -50.4318) -> (2.5283, -50.4318)
  line L273 (2.5283, -50.4318) -> (4.4201, -50.4318)
  line L274 (4.4201, -50.4318) -> (4.4201, -51.0052)
  line L275 (4.4201, -51.0052) -> (4.4201, -51.5782)
  line L276 (4.4201, -51.5782) -> (0.1014, -51.5782)
  line L277 (0.1014, -51.5782) -> (-4.217, -51.5782)
  line L278 (-4.217, -51.5782) -> (-4.217, -51.0052)
  line L279 (-4.217, -51.0052) -> (-4.217, -50.4318)
  line L280 (-4.217, -50.4318) -> (-2.3445, -50.4318)
  spline S375 degree 3 poles (-4.1242, -23.1828) (-3.7685, -21.9036) (-2.8202, -21.182) (-1.5036, -21.1892) knots 0 0 0 0 1 1 1 1
  spline S376 degree 3 poles (-1.5036, -21.1892) (-0.1456, -21.1967) (0.6599, -21.8922) (0.9275, -23.2887) knots 0 0 0 0 1 1 1 1
  spline S377 degree 3 poles (0.9275, -23.2887) (0.9891, -23.6089) (1.0032, -23.6412) (1.0813, -23.6412) knots 0 0 0 0 1 1 1 1
  spline S378 degree 3 poles (1.0813, -23.6412) (1.1336, -23.6412) (1.7947, -23.1848) (2.7698, -22.4756) knots 0 0 0 0 1 1 1 1
  spline S379 degree 3 poles (2.7698, -22.4756) (3.651, -21.8344) (4.383, -21.3099) (4.396, -21.3099) knots 0 0 0 0 1 1 1 1
  spline S380 degree 3 poles (4.396, -21.3099) (4.4094, -21.3099) (4.4201, -21.6418) (4.4201, -22.0477) knots 0 0 0 0 1 1 1 1
  line L281 (4.4201, -22.0477) -> (4.4201, -22.7851)
  line L282 (4.4201, -22.7851) -> (2.7203, -23.9491)
  line L283 (2.7203, -23.9491) -> (1.0204, -25.1127)
  line L284 (1.0204, -25.1127) -> (1.0194, -25.6572)
  line L285 (1.0194, -25.6572) -> (1.0187, -26.2017)
  line L286 (1.0187, -26.2017) -> (2.7192, -26.2017)
  line L287 (2.7192, -26.2017) -> (4.4201, -26.2017)
  line L288 (4.4201, -26.2017) -> (4.4201, -26.7751)
  line L289 (4.4201, -26.7751) -> (4.4201, -27.3484)
  line L290 (4.4201, -27.3484) -> (0.0989, -27.3484)
  line L291 (0.0989, -27.3484) -> (-4.2222, -27.3484)
  line L292 (-4.2222, -27.3484) -> (-4.2078, -25.3896)
  spline S381 degree 3 poles (-4.2078, -25.3896) (-4.1947, -23.6471) (-4.1854, -23.4036) (-4.1242, -23.1828) knots 0 0 0 0 1 1 1 1
  spline S382 degree 3 poles (-4.0905, -3.7887) (-3.4607, -2.0063) (-1.1661, -1.6854) (-0.1848, -3.2425) knots 0 0 0 0 1 1 1 1
  spline S383 degree 3 poles (-0.1848, -3.2425) (-0.0314, -3.486) (0.0487, -3.4819) (0.2042, -3.2235) knots 0 0 0 0 1 1 1 1
  spline S384 degree 3 poles (0.2042, -3.2235) (1.3324, -1.349) (3.748, -1.4776) (4.3283, -3.4433) knots 0 0 0 0 1 1 1 1
  spline S385 degree 3 poles (4.3283, -3.4433) (4.3881, -3.647) (4.3974, -3.8991) (4.4101, -5.7076) knots 0 0 0 0 1 1 1 1
  line L293 (4.4101, -5.7076) -> (4.4242, -7.7428)
  line L294 (4.4242, -7.7428) -> (0.1017, -7.7428)
  line L295 (0.1017, -7.7428) -> (-4.2212, -7.7428)
  line L296 (-4.2212, -7.7428) -> (-4.2095, -5.9178)
  line L297 (-4.2095, -5.9178) -> (-4.1981, -4.0931)
  line L298 (-4.1981, -4.0931) -> (-4.0905, -3.7887)
  line L299 (-3.644, 15.7227) -> (-3.0706, 15.7227)
  line L300 (-3.0706, 15.7227) -> (-3.0706, 14.6338)
  line L301 (-3.0706, 14.6338) -> (-3.0706, 13.5444)
  line L302 (-3.0706, 13.5444) -> (0.6747, 13.5444)
  line L303 (0.6747, 13.5444) -> (4.4201, 13.5444)
  line L304 (4.4201, 13.5444) -> (4.4201, 12.9711)
  line L305 (4.4201, 12.9711) -> (4.4201, 12.398)
  line L306 (4.4201, 12.398) -> (0.6747, 12.398)
  line L307 (0.6747, 12.398) -> (-3.0706, 12.398)
  line L308 (-3.0706, 12.398) -> (-3.0706, 11.328)
  line L309 (-3.0706, 11.328) -> (-3.0706, 10.2579)
  line L310 (-3.0706, 10.2579) -> (-3.644, 10.2579)
  line L311 (-3.644, 10.2579) -> (-4.217, 10.2579)
  line L312 (-4.217, 10.2579) -> (-4.217, 12.9903)
  line L313 (-4.217, 12.9903) -> (-4.217, 15.7227)
  line L314 (-4.217, 15.7227) -> (-3.644, 15.7227)
  line L315 (0.1014, 18.7038) -> (4.4201, 18.7038)
  line L316 (4.4201, 18.7038) -> (4.4201, 18.1304)
  line L317 (4.4201, 18.1304) -> (4.4201, 17.5574)
  line L318 (4.4201, 17.5574) -> (0.1014, 17.5574)
  line L319 (0.1014, 17.5574) -> (-4.217, 17.5574)
  line L320 (-4.217, 17.5574) -> (-4.217, 18.1304)
  line L321 (-4.217, 18.1304) -> (-4.217, 18.7038)
  line L322 (-4.217, 18.7038) -> (0.1014, 18.7038)
  spline S386 degree 3 poles (-3.1601, -78.8841) (-2.8178, -80.4814) (-1.6085, -81.4108) (0.1206, -81.4046) knots 0 0 0 0 1 1 1 1
  spline S387 degree 3 poles (0.1206, -81.4046) (2.409, -81.3967) (3.8753, -79.551) (3.4044, -77.2709) knots 0 0 0 0 1 1 1 1
  spline S388 degree 3 poles (3.4044, -77.2709) (2.7285, -73.9992) (-2.0525, -73.7092) (-3.0637, -76.8784) knots 0 0 0 0 1 1 1 1
  spline S389 degree 3 poles (-3.0637, -76.8784) (-3.2347, -77.4136) (-3.2787, -78.3306) (-3.1601, -78.8841) knots 0 0 0 0 1 1 1 1
  spline S390 degree 3 poles (-3.1601, -38.3352) (-2.8178, -39.9325) (-1.6085, -40.8619) (0.1206, -40.856) knots 0 0 0 0 1 1 1 1
  spline S391 degree 3 poles (0.1206, -40.856) (2.409, -40.8478) (3.8753, -39.0021) (3.4044, -36.722) knots 0 0 0 0 1 1 1 1
  spline S392 degree 3 poles (3.4044, -36.722) (2.7285, -33.4503) (-2.0525, -33.1603) (-3.0637, -36.3295) knots 0 0 0 0 1 1 1 1
  spline S393 degree 3 poles (-3.0637, -36.3295) (-3.2347, -36.8651) (-3.2787, -37.7817) (-3.1601, -38.3352) knots 0 0 0 0 1 1 1 1
  spline S394 degree 3 poles (-3.1601, -15.4812) (-2.8178, -17.0785) (-1.6085, -18.0079) (0.1206, -18.0017) knots 0 0 0 0 1 1 1 1
  spline S395 degree 3 poles (0.1206, -18.0017) (2.409, -17.9938) (3.8753, -16.1478) (3.4044, -13.868) knots 0 0 0 0 1 1 1 1
  spline S396 degree 3 poles (3.4044, -13.868) (2.7285, -10.5963) (-2.0525, -10.306) (-3.0637, -13.4752) knots 0 0 0 0 1 1 1 1
  spline S397 degree 3 poles (-3.0637, -13.4752) (-3.2347, -14.0108) (-3.2787, -14.9274) (-3.1601, -15.4812) knots 0 0 0 0 1 1 1 1
  spline S398 degree 3 poles (-3.1601, 3.6278) (-2.8178, 2.0304) (-1.6085, 1.101) (0.1206, 1.1069) knots 0 0 0 0 1 1 1 1
  spline S399 degree 3 poles (0.1206, 1.1069) (2.409, 1.1152) (3.8753, 2.9608) (3.4044, 5.2409) knots 0 0 0 0 1 1 1 1
  spline S400 degree 3 poles (3.4044, 5.2409) (2.7285, 8.5127) (-2.0525, 8.8026) (-3.0637, 5.6334) knots 0 0 0 0 1 1 1 1
  spline S401 degree 3 poles (-3.0637, 5.6334) (-3.2347, 5.0978) (-3.2787, 4.1812) (-3.1601, 3.6278) knots 0 0 0 0 1 1 1 1
  line L323 (-1.6188, -89.6049) -> (-0.0861, -89.6049)
  line L324 (-0.0861, -89.6049) -> (-0.0975, -88.1431)
  line L325 (-0.0975, -88.1431) -> (-0.1088, -86.6812)
  line L326 (-0.1088, -86.6812) -> (-0.2137, -86.4821)
  spline S402 degree 3 poles (-0.2137, -86.4821) (-0.7998, -85.3704) (-2.4522, -85.3835) (-3.0042, -86.5041) knots 0 0 0 0 1 1 1 1
  line L327 (-3.0042, -86.5041) -> (-3.1281, -86.7559)
  line L328 (-3.1281, -86.7559) -> (-3.1398, -88.1802)
  line L329 (-3.1398, -88.1802) -> (-3.1515, -89.6049)
  line L330 (-3.1515, -89.6049) -> (-1.6188, -89.6049)
  line L331 (-1.6188, -26.2017) -> (-0.0861, -26.2017)
  line L332 (-0.0861, -26.2017) -> (-0.0975, -24.7399)
  line L333 (-0.0975, -24.7399) -> (-0.1088, -23.278)
  line L334 (-0.1088, -23.278) -> (-0.2137, -23.0789)
  spline S403 degree 3 poles (-0.2137, -23.0789) (-0.7998, -21.9672) (-2.4522, -21.9806) (-3.0042, -23.1012) knots 0 0 0 0 1 1 1 1
  line L335 (-3.0042, -23.1012) -> (-3.1281, -23.3527)
  line L336 (-3.1281, -23.3527) -> (-3.1398, -24.7773)
  line L337 (-3.1398, -24.7773) -> (-3.1515, -26.2017)
  line L338 (-3.1515, -26.2017) -> (-1.6188, -26.2017)
  line L339 (-1.7691, -97.3629) -> (-0.4294, -97.3629)
  line L340 (-0.4294, -97.3629) -> (-0.4411, -96.245)
  line L341 (-0.4411, -96.245) -> (-0.4528, -95.1271)
  line L342 (-0.4528, -95.1271) -> (-0.5542, -94.9104)
  spline S404 degree 3 poles (-0.5542, -94.9104) (-1.0344, -93.8865) (-2.4319, -93.8456) (-2.9382, -94.8406) knots 0 0 0 0 1 1 1 1
  spline S405 degree 3 poles (-2.9382, -94.8406) (-3.0864, -95.132) (-3.1078, -95.3249) (-3.1085, -96.3599) knots 0 0 0 0 1 1 1 1
  line L343 (-3.1085, -96.3599) -> (-3.1088, -97.3629)
  line L344 (-3.1088, -97.3629) -> (-1.7691, -97.3629)
  line L345 (-1.7691, -6.6346) -> (-0.4294, -6.6346)
  line L346 (-0.4294, -6.6346) -> (-0.4411, -5.5167)
  line L347 (-0.4411, -5.5167) -> (-0.4528, -4.3988)
  line L348 (-0.4528, -4.3988) -> (-0.5542, -4.1818)
  spline S406 degree 3 poles (-0.5542, -4.1818) (-1.0344, -3.1578) (-2.4319, -3.1173) (-2.9382, -4.112) knots 0 0 0 0 1 1 1 1
  spline S407 degree 3 poles (-2.9382, -4.112) (-3.0864, -4.4033) (-3.1078, -4.5963) (-3.1085, -5.6313) knots 0 0 0 0 1 1 1 1
  line L349 (-3.1085, -5.6313) -> (-3.1088, -6.6346)
  line L350 (-3.1088, -6.6346) -> (-1.7691, -6.6346)
  spline S408 degree 3 poles (-2.6479, -77.2613) (-1.9445, -74.7259) (1.955, -74.619) (2.7918, -77.1116) knots 0 0 0 0 1 1 1 1
  spline S409 degree 3 poles (2.7918, -77.1116) (3.4343, -79.0251) (2.1135, -80.8051) (0.0632, -80.7896) knots 0 0 0 0 1 1 1 1
  spline S410 degree 3 poles (0.0632, -80.7896) (-1.8884, -80.7748) (-3.1628, -79.1162) (-2.6479, -77.2613) knots 0 0 0 0 1 1 1 1
  spline S411 degree 3 poles (-2.6479, -36.7124) (-1.9445, -34.1774) (1.955, -34.0701) (2.7918, -36.5627) knots 0 0 0 0 1 1 1 1
  spline S412 degree 3 poles (2.7918, -36.5627) (3.4343, -38.4762) (2.1135, -40.2565) (0.0632, -40.2407) knots 0 0 0 0 1 1 1 1
  spline S413 degree 3 poles (0.0632, -40.2407) (-1.8884, -40.2259) (-3.1628, -38.5673) (-2.6479, -36.7124) knots 0 0 0 0 1 1 1 1
  spline S414 degree 3 poles (-2.6479, -13.858) (-1.9445, -11.3231) (1.955, -11.2158) (2.7918, -13.7084) knots 0 0 0 0 1 1 1 1
  spline S415 degree 3 poles (2.7918, -13.7084) (3.4343, -15.6219) (2.1135, -17.4022) (0.0632, -17.3867) knots 0 0 0 0 1 1 1 1
  spline S416 degree 3 poles (0.0632, -17.3867) (-1.8884, -17.3719) (-3.1628, -15.7134) (-2.6479, -13.858) knots 0 0 0 0 1 1 1 1
  spline S417 degree 3 poles (-2.6479, 5.2506) (-1.9445, 7.7855) (1.955, 7.8928) (2.7918, 5.4002) knots 0 0 0 0 1 1 1 1
  spline S418 degree 3 poles (2.7918, 5.4002) (3.4343, 3.4867) (2.1135, 1.7064) (0.0632, 1.7222) knots 0 0 0 0 1 1 1 1
  spline S419 degree 3 poles (0.0632, 1.7222) (-1.8884, 1.737) (-3.1628, 3.3956) (-2.6479, 5.2506) knots 0 0 0 0 1 1 1 1
  spline S420 degree 3 poles (-2.6379, -87.0187) (-2.4398, -86.2558) (-1.3433, -86.0339) (-0.7812, -86.6434) knots 0 0 0 0 1 1 1 1
  spline S421 degree 3 poles (-0.7812, -86.6434) (-0.5659, -86.8773) (-0.5487, -86.9801) (-0.5484, -88.0474) knots 0 0 0 0 1 1 1 1
  line L351 (-0.5484, -88.0474) -> (-0.5484, -88.9933)
  line L352 (-0.5484, -88.9933) -> (-1.6184, -88.9933)
  line L353 (-1.6184, -88.9933) -> (-2.6885, -88.9933)
  line L354 (-2.6885, -88.9933) -> (-2.6885, -88.1035)
  spline S422 degree 3 poles (-2.6885, -88.1035) (-2.6885, -87.4892) (-2.6727, -87.1535) (-2.6379, -87.0187) knots 0 0 0 0 1 1 1 1
  spline S423 degree 3 poles (-2.6379, -23.6158) (-2.4398, -22.8526) (-1.3433, -22.6307) (-0.7812, -23.2402) knots 0 0 0 0 1 1 1 1
  spline S424 degree 3 poles (-0.7812, -23.2402) (-0.5659, -23.4741) (-0.5487, -23.5769) (-0.5484, -24.6446) knots 0 0 0 0 1 1 1 1
  line L355 (-0.5484, -24.6446) -> (-0.5484, -25.5905)
  line L356 (-0.5484, -25.5905) -> (-1.6184, -25.5905)
  line L357 (-1.6184, -25.5905) -> (-2.6885, -25.5905)
  line L358 (-2.6885, -25.5905) -> (-2.6885, -24.7006)
  spline S425 degree 3 poles (-2.6885, -24.7006) (-2.6885, -24.0863) (-2.6727, -23.7503) (-2.6379, -23.6158) knots 0 0 0 0 1 1 1 1
  spline S426 degree 3 poles (-2.5595, -95.2802) (-2.3057, -94.6948) (-1.5483, -94.5713) (-1.1149, -95.0449) knots 0 0 0 0 1 1 1 1
  spline S427 degree 3 poles (-1.1149, -95.0449) (-0.9381, -95.2382) (-0.8923, -95.4646) (-0.8923, -96.147) knots 0 0 0 0 1 1 1 1
  line L359 (-0.8923, -96.147) -> (-0.8923, -96.7517)
  line L360 (-0.8923, -96.7517) -> (-1.7756, -96.7517)
  line L361 (-1.7756, -96.7517) -> (-2.6589, -96.7517)
  line L362 (-2.6589, -96.7517) -> (-2.6424, -96.0923)
  spline S428 degree 3 poles (-2.6424, -96.0923) (-2.6297, -95.5781) (-2.6114, -95.3992) (-2.5595, -95.2802) knots 0 0 0 0 1 1 1 1
  spline S429 degree 3 poles (-2.5595, -4.5516) (-2.3057, -3.9661) (-1.5483, -3.843) (-1.1149, -4.3163) knots 0 0 0 0 1 1 1 1
  spline S430 degree 3 poles (-1.1149, -4.3163) (-0.9381, -4.5096) (-0.8923, -4.7359) (-0.8923, -5.4183) knots 0 0 0 0 1 1 1 1
  line L363 (-0.8923, -5.4183) -> (-0.8923, -6.023)
  line L364 (-0.8923, -6.023) -> (-1.7756, -6.023)
  line L365 (-1.7756, -6.023) -> (-2.6589, -6.023)
  line L366 (-2.6589, -6.023) -> (-2.6424, -5.3636)
  spline S431 degree 3 poles (-2.6424, -5.3636) (-2.6297, -4.8494) (-2.6114, -4.6709) (-2.5595, -4.5516) knots 0 0 0 0 1 1 1 1
  line L367 (1.955, -97.3629) -> (3.2389, -97.3629)
  line L368 (3.2389, -97.3629) -> (3.2276, -96.0923)
  line L369 (3.2276, -96.0923) -> (3.2162, -94.8214)
  line L370 (3.2162, -94.8214) -> (3.1062, -94.5833)
  spline S432 degree 3 poles (3.1062, -94.5833) (2.6501, -93.5958) (1.267, -93.6189) (0.8037, -94.6219) knots 0 0 0 0 1 1 1 1
  line L371 (0.8037, -94.6219) -> (0.6937, -94.8599)
  line L372 (0.6937, -94.8599) -> (0.6823, -96.1112)
  line L373 (0.6823, -96.1112) -> (0.671, -97.3629)
  line L374 (0.671, -97.3629) -> (1.955, -97.3629)
  line L375 (1.955, -6.6346) -> (3.2389, -6.6346)
  line L376 (3.2389, -6.6346) -> (3.2276, -5.3636)
  line L377 (3.2276, -5.3636) -> (3.2162, -4.0931)
  line L378 (3.2162, -4.0931) -> (3.1062, -3.8547)
  spline S433 degree 3 poles (3.1062, -3.8547) (2.6501, -2.8672) (1.267, -2.8906) (0.8037, -3.8932) knots 0 0 0 0 1 1 1 1
  line L379 (0.8037, -3.8932) -> (0.6937, -4.1313)
  line L380 (0.6937, -4.1313) -> (0.6823, -5.3829)
  line L381 (0.6823, -5.3829) -> (0.671, -6.6346)
  line L382 (0.671, -6.6346) -> (1.955, -6.6346)
  spline S434 degree 3 poles (1.224, -94.9552) (1.4514, -94.5276) (1.913, -94.3677) (2.3336, -94.5713) knots 0 0 0 0 1 1 1 1
  spline S435 degree 3 poles (2.3336, -94.5713) (2.7058, -94.7515) (2.7767, -94.9786) (2.7767, -95.9932) knots 0 0 0 0 1 1 1 1
  line L383 (2.7767, -95.9932) -> (2.7767, -96.7517)
  line L384 (2.7767, -96.7517) -> (1.9519, -96.7517)
  line L385 (1.9519, -96.7517) -> (1.1267, -96.7517)
  line L386 (1.1267, -96.7517) -> (1.1398, -95.9203)
  spline S436 degree 3 poles (1.1398, -95.9203) (1.1511, -95.199) (1.1621, -95.0714) (1.224, -94.9552) knots 0 0 0 0 1 1 1 1
  spline S437 degree 3 poles (1.224, -4.2269) (1.4514, -3.799) (1.913, -3.6394) (2.3336, -3.8427) knots 0 0 0 0 1 1 1 1
  spline S438 degree 3 poles (2.3336, -3.8427) (2.7058, -4.0232) (2.7767, -4.2499) (2.7767, -5.2646) knots 0 0 0 0 1 1 1 1
  line L387 (2.7767, -5.2646) -> (2.7767, -6.023)
  line L388 (2.7767, -6.023) -> (1.9519, -6.023)
  line L389 (1.9519, -6.023) -> (1.1267, -6.023)
  line L390 (1.1267, -6.023) -> (1.1398, -5.1917)
  spline S439 degree 3 poles (1.1398, -5.1917) (1.1511, -4.4707) (1.1621, -4.3428) (1.224, -4.2269) knots 0 0 0 0 1 1 1 1
  spline S440 degree 3 poles (8.4736, -39.2274) (8.6081, -40.252) (9.5217, -41.1449) (10.4352, -41.1449) knots 0 0 0 0 1 1 1 1
  line L391 (10.4352, -41.1449) -> (10.5732, -41.1449)
  line L392 (10.5732, -41.1449) -> (10.5732, -40.4237)
  line L393 (10.5732, -40.4237) -> (10.5732, -39.7027)
  line L394 (10.5732, -39.7027) -> (10.4346, -39.68)
  spline S441 degree 3 poles (10.4346, -39.68) (9.6194, -39.5479) (9.6335, -38.3221) (10.4524, -38.1456) knots 0 0 0 0 1 1 1 1
  spline S442 degree 3 poles (10.4524, -38.1456) (10.8304, -38.0641) (10.7613, -38.0094) (12.5523, -39.8104) knots 0 0 0 0 1 1 1 1
  spline S443 degree 3 poles (12.5523, -39.8104) (13.9175, -41.1831) (14.2019, -41.4514) (14.2896, -41.4511) knots 0 0 0 0 1 1 1 1
  line L395 (14.2896, -41.4511) -> (14.3949, -41.4507)
  line L396 (14.3949, -41.4507) -> (14.3949, -39.0619)
  line L397 (14.3949, -39.0619) -> (14.3949, -36.6735)
  line L398 (14.3949, -36.6735) -> (13.7641, -36.6735)
  line L399 (13.7641, -36.6735) -> (13.1336, -36.6735)
  line L400 (13.1336, -36.6735) -> (13.1336, -37.5224)
  line L401 (13.1336, -37.5224) -> (13.1336, -38.3709)
  line L402 (13.1336, -38.3709) -> (12.5317, -37.7748)
  spline S444 degree 3 poles (12.5317, -37.7748) (11.6546, -36.9063) (11.2728, -36.6962) (10.5732, -36.6972) knots 0 0 0 0 1 1 1 1
  spline S445 degree 3 poles (10.5732, -36.6972) (9.2696, -36.6996) (8.2958, -37.8729) (8.4736, -39.2274) knots 0 0 0 0 1 1 1 1
  spline S446 degree 3 poles (8.475, -33.9861) (8.5933, -35.0118) (9.3232, -35.8476) (10.3211, -36.1001) knots 0 0 0 0 1 1 1 1
  spline S447 degree 3 poles (10.3211, -36.1001) (10.709, -36.1981) (12.2562, -36.2116) (12.6871, -36.1201) knots 0 0 0 0 1 1 1 1
  spline S448 degree 3 poles (12.6871, -36.1201) (15.1898, -35.5897) (15.2255, -31.7466) (12.7339, -31.1134) knots 0 0 0 0 1 1 1 1
  spline S449 degree 3 poles (12.7339, -31.1134) (12.3514, -31.0161) (10.6409, -31.0308) (10.2667, -31.1347) knots 0 0 0 0 1 1 1 1
  spline S450 degree 3 poles (10.2667, -31.1347) (9.0684, -31.4666) (8.3216, -32.655) (8.475, -33.9861) knots 0 0 0 0 1 1 1 1
  spline S451 degree 3 poles (8.4736, -28.4883) (8.6081, -29.513) (9.5217, -30.4059) (10.4352, -30.4059) knots 0 0 0 0 1 1 1 1
  line L403 (10.4352, -30.4059) -> (10.5732, -30.4059)
  line L404 (10.5732, -30.4059) -> (10.5732, -29.6846)
  line L405 (10.5732, -29.6846) -> (10.5732, -28.9637)
  line L406 (10.5732, -28.9637) -> (10.4346, -28.941)
  spline S452 degree 3 poles (10.4346, -28.941) (9.6194, -28.8089) (9.6335, -27.583) (10.4524, -27.4066) knots 0 0 0 0 1 1 1 1
  spline S453 degree 3 poles (10.4524, -27.4066) (10.8304, -27.325) (10.7613, -27.27) (12.5523, -29.0713) knots 0 0 0 0 1 1 1 1
  spline S454 degree 3 poles (12.5523, -29.0713) (13.9175, -30.4441) (14.2019, -30.7123) (14.2896, -30.712) knots 0 0 0 0 1 1 1 1
  line L407 (14.2896, -30.712) -> (14.3949, -30.7117)
  line L408 (14.3949, -30.7117) -> (14.3949, -28.3229)
  line L409 (14.3949, -28.3229) -> (14.3949, -25.9344)
  line L410 (14.3949, -25.9344) -> (13.7641, -25.9344)
  line L411 (13.7641, -25.9344) -> (13.1336, -25.9344)
  line L412 (13.1336, -25.9344) -> (13.1336, -26.783)
  line L413 (13.1336, -26.783) -> (13.1336, -27.6319)
  line L414 (13.1336, -27.6319) -> (12.5317, -27.0358)
  spline S455 degree 3 poles (12.5317, -27.0358) (11.6546, -26.1669) (11.2728, -25.9571) (10.5732, -25.9582) knots 0 0 0 0 1 1 1 1
  spline S456 degree 3 poles (10.5732, -25.9582) (9.2696, -25.9602) (8.2958, -27.1338) (8.4736, -28.4883) knots 0 0 0 0 1 1 1 1
  spline S457 degree 3 poles (8.4716, -23.5972) (8.5947, -24.4234) (9.2692, -25.0855) (10.0283, -25.1254) knots 0 0 0 0 1 1 1 1
  line L415 (10.0283, -25.1254) -> (10.3056, -25.1402)
  line L416 (10.3056, -25.1402) -> (10.3056, -24.4337)
  line L417 (10.3056, -24.4337) -> (10.3056, -23.7276)
  line L418 (10.3056, -23.7276) -> (10.1487, -23.7025)
  spline S458 degree 3 poles (10.1487, -23.7025) (9.7834, -23.644) (9.6514, -23.2942) (9.9004, -23.0452) knots 0 0 0 0 1 1 1 1
  spline S459 degree 3 poles (9.9004, -23.0452) (10.2206, -22.7249) (10.6877, -23.0087) (10.6877, -23.5229) knots 0 0 0 0 1 1 1 1
  line L419 (10.6877, -23.5229) -> (10.6877, -23.7176)
  line L420 (10.6877, -23.7176) -> (11.3564, -23.7176)
  line L421 (11.3564, -23.7176) -> (12.0254, -23.7176)
  line L422 (12.0254, -23.7176) -> (12.0257, -23.4596)
  spline S460 degree 3 poles (12.0257, -23.4596) (12.0261, -22.8698) (12.3184, -22.5413) (12.7676, -22.6255) knots 0 0 0 0 1 1 1 1
  spline S461 degree 3 poles (12.7676, -22.6255) (13.5264, -22.7676) (13.428, -24.0279) (12.6531, -24.0922) knots 0 0 0 0 1 1 1 1